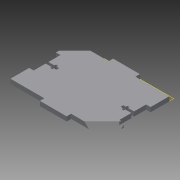
# Autodesk Inventor part: back
Saved by Autodesk Inventor 2014 (Build 180170000, 170)
## iProperties
Created: 2014-03-02
Part Number: back
Material: 常规
Document SubType Name: Modeling
Designer: Keshuai
Density: 1 g/cm^3
Appearance: 默认
Author: Keshuai
Autodesk Inventor part; units mm, degrees
ref_plane "YZ Plane" through (0, 0, 0) normal (1, 0, 0) x (0, 1, 0)
sketch "slot" plane through (0, 0, 0) normal (0, 0, 1) x (1, 0, 0)
  line L0 (-18.25, 14.2) -> (-11.75, 11.8) construction
  line L1 (-11.75, 14.2) -> (-18.25, 11.8) construction
  line L2 (-18.25, 14.2) -> (-16.5, 14.2)
  line L3 (-13.5, 14.2) -> (-11.75, 14.2)
  line L4 (-16.5, 9) -> (-16.5, 11.8)
  line L5 (-16.5, 14.2) -> (-16.5, 21)
  line L6 (-13.5, 21) -> (-13.5, 14.2)
  line L7 (-13.5, 11.8) -> (-13.5, 9)
  line L8 (-11.75, 11.8) -> (-13.5, 11.8)
  line L9 (-16.5, 11.8) -> (-18.25, 11.8)
  line L10 (-16.5, 21) -> (-13.5, 21)
  line L11 (-13.5, 9) -> (-16.5, 9)
  line L12 (-11.75, 14.2) -> (-11.75, 11.8)
  line L13 (-18.25, 11.8) -> (-18.25, 14.2)
  point P0 (-15, 21)
  point P1 (-15, 13)
  dimension "d8" = 3
  dimension "d9" = 12
  dimension "d10" = 6.5
  dimension "d11" = 2.4
  dimension "d12" = 8
  measures "d8" distance of L7.end L4.start
  measures "d9" distance of L6.start L7.end
  measures "d10" distance of L0.end L1.end
  measures "d11" distance of L1.start L0.end
  measures "d12" distance from line of L10 point (-15, 13)
ref_plane "工作平面1" through (0, 0, 0) normal (0, 0, 1) x (1, 0, 0)
sketch "草图2" plane through (0, 0, 0) normal (0, 0, 1) x (1, 0, 0)
  line L0 (74, -10) -> (74, -69) projected
  line L1 (74, -69) -> (69, -69) projected
  line L2 (69, -69) -> (69, -10) projected
  line L3 (69, -10) -> (74, -10) projected
  circle A0 centre (48, 2.5) radius 1.5 projected
  circle A1 centre (48, -74.5) radius 1.5 projected
  line L4 (33, -77) -> (33, -72) projected
  line L5 (63, -77) -> (33, -77) projected
  line L6 (63, -72) -> (63, -77) projected
  line L7 (96, -72) -> (63, -72) projected
  line L8 (96, 0) -> (96, -72) projected
  line L9 (63, 0) -> (96, 0) projected
  line L10 (63, 5) -> (63, 0) projected
  line L11 (33, 5) -> (63, 5) projected
  line L12 (33, 0) -> (33, 5) projected
  line L13 (0, 0) -> (33, 0) projected
  line L14 (0, -72) -> (0, 0) projected
  line L15 (33, -72) -> (0, -72) projected
extrude "拉伸2" add sketch "草图2" along normal blind 5 contours L0 L1 L2 L3 | A0 | A1 | L4 L15 L14 L13 L12 L11 L10 L9 L8 L7 L6 L5
sketch "草图3" plane through (0, -72, 0) normal (-1, 0, 0) x (0, 0, 1)
  line L0 (0, 0) -> (0, 72) projected
  line L1 (0, 0) -> (5, 0) projected
  line L2 (5, 72) -> (5, 0) projected
  line L3 (0, 72) -> (5, 72) projected
  circle A0 centre (2.5, 36) radius 1.5 projected
  circle A1 centre (-35, -2.5) radius 1.5 projected
  circle A2 centre (-85, -2.5) radius 1.5 projected
  circle A3 centre (-85, 74.5) radius 1.5 projected
  circle A4 centre (-35, 74.5) radius 1.5 projected
  line L4 (-20, 0) -> (-20, -5) projected
  line L5 (0, 0) -> (-20, 0) projected
  line L6 (0, 21) -> (0, 0) projected
  line L7 (0, 21) -> (5, 21) projected
  line L8 (5, 21) -> (5, 51) projected
  line L9 (5, 51) -> (0, 51) projected
  line L10 (0, 72) -> (0, 51) projected
  line L11 (-20, 72) -> (0, 72) projected
  line L12 (-20, 77) -> (-20, 72) projected
  line L13 (-50, 77) -> (-20, 77) projected
  line L14 (-50, 72) -> (-50, 77) projected
  line L15 (-70, 72) -> (-50, 72) projected
  line L16 (-70, 77) -> (-70, 72) projected
  line L17 (-100, 77) -> (-70, 77) projected
  line L18 (-100, 72) -> (-100, 77) projected
  line L19 (-121, 72) -> (-100, 72) projected
  line L20 (-121, 0) -> (-121, 72) projected
  line L21 (-100, 0) -> (-121, 0) projected
  line L22 (-100, -5) -> (-100, 0) projected
  line L23 (-70, -5) -> (-100, -5) projected
  line L24 (-70, 0) -> (-70, -5) projected
  line L25 (-50, 0) -> (-70, 0) projected
  line L26 (-50, -5) -> (-50, 0) projected
  line L27 (-20, -5) -> (-50, -5) projected
ref_plane "工作平面2" through (-5, -77, -121) normal (-1, 0, 0) x (0, 0, 1)
extrude "拉伸3" add sketch "草图3" along normal up to surface (5 mm away) contours L0 L7 L2 L1 | L0 L3 L2 L9
sketch "草图4" plane through (96, -72, 0) normal (1, 0, 0) x (0, 0, -1)
  line L0 (0, 72) -> (0, 0) projected
  line L1 (0, 72) -> (-5, 72) projected
  line L2 (-5, 0) -> (-5, 72) projected
  line L3 (0, 0) -> (-5, 0) projected
  circle A0 centre (-2.5, 36) radius 1.5 projected
  circle A1 centre (35, -2.5) radius 1.5 projected
  circle A2 centre (85, -2.5) radius 1.5 projected
  circle A3 centre (85, 74.5) radius 1.5 projected
  circle A4 centre (35, 74.5) radius 1.5 projected
  line L4 (20, 0) -> (20, -5) projected
  line L5 (20, -5) -> (50, -5) projected
  line L6 (50, -5) -> (50, 0) projected
  line L7 (50, 0) -> (70, 0) projected
  line L8 (70, 0) -> (70, -5) projected
  line L9 (70, -5) -> (100, -5) projected
  line L10 (100, -5) -> (100, 0) projected
  line L11 (100, 0) -> (121, 0) projected
  line L12 (121, 0) -> (121, 72) projected
  line L13 (121, 72) -> (100, 72) projected
  line L14 (100, 72) -> (100, 77) projected
  line L15 (100, 77) -> (70, 77) projected
  line L16 (70, 77) -> (70, 72) projected
  line L17 (70, 72) -> (50, 72) projected
  line L18 (50, 72) -> (50, 77) projected
  line L19 (50, 77) -> (20, 77) projected
  line L20 (20, 77) -> (20, 72) projected
  line L21 (20, 72) -> (0, 72) projected
  line L22 (0, 72) -> (0, 51) projected
  line L23 (0, 51) -> (-5, 51) projected
  line L24 (-5, 51) -> (-5, 21) projected
  line L25 (-5, 21) -> (0, 21) projected
  line L26 (0, 21) -> (0, 0) projected
  line L27 (0, 0) -> (20, 0) projected
ref_plane "工作平面3" through (101, -77, -121) normal (1, 0, 0) x (0, 1, 0)
extrude "拉伸4" add sketch "草图4" along normal up to surface (5 mm away) contours L0 L23 L2 L1 | L0 L3 L2 L25
sketch "草图5" plane through (0, 0, 5) normal (0, 0, 1) x (1, 0, 0)
  line L0 (0, -21) -> (0, -51) projected
  line L1 (96, -51) -> (96, -21) projected
  line L2 (-5, -37.5) -> (-5, -34.5) projected
  line L3 (101, -34.5) -> (101, -37.5) projected
  line L4 (6.8, -39.25) -> (9.2, -32.75) construction
  line L5 (6.8, -32.75) -> (9.2, -39.25) construction
  line L6 (6.8, -39.25) -> (6.8, -37.5)
  line L7 (6.8, -34.5) -> (6.8, -32.75)
  line L8 (12, -37.5) -> (9.2, -37.5)
  line L9 (6.8, -37.5) -> (0, -37.5)
  line L10 (0, -34.5) -> (6.8, -34.5)
  line L11 (9.2, -34.5) -> (12, -34.5)
  line L12 (9.2, -32.75) -> (9.2, -34.5)
  line L13 (9.2, -37.5) -> (9.2, -39.25)
  line L14 (0, -37.5) -> (0, -34.5)
  line L15 (12, -34.5) -> (12, -37.5)
  line L16 (6.8, -32.75) -> (9.2, -32.75)
  line L17 (9.2, -39.25) -> (6.8, -39.25)
  line L18 (89.2, -32.75) -> (86.8, -39.25) construction
  line L19 (89.2, -39.25) -> (86.8, -32.75) construction
  line L20 (89.2, -32.75) -> (89.2, -34.5)
  line L21 (89.2, -37.5) -> (89.2, -39.25)
  line L22 (84, -34.5) -> (86.8, -34.5)
  line L23 (89.2, -34.5) -> (96, -34.5)
  line L24 (96, -37.5) -> (89.2, -37.5)
  line L25 (86.8, -37.5) -> (84, -37.5)
  line L26 (86.8, -39.25) -> (86.8, -37.5)
  line L27 (86.8, -34.5) -> (86.8, -32.75)
  line L28 (96, -34.5) -> (96, -37.5)
  line L29 (84, -37.5) -> (84, -34.5)
  line L30 (89.2, -39.25) -> (86.8, -39.25)
  line L31 (86.8, -32.75) -> (89.2, -32.75)
  point P0 (0, 0)
  constraints: 2 vertical
extrude "拉伸5" cut sketch "草图5" against normal through all
